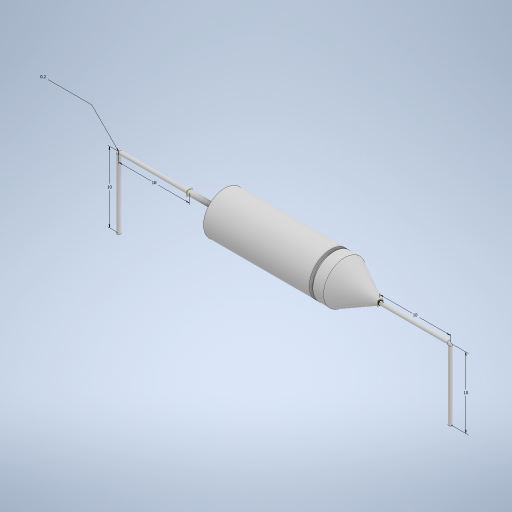
# Autodesk Inventor part: k50-29
Saved by Autodesk Inventor 2024 (Build 280153000, 153)
## iProperties
Created: 2023-12-15
Part Number: k50-29
Material: Generic
Document SubType Name: Sheet Metal
Designer: user
Density: 1 g/cm^3
Sheet Metal Rule: Default
Appearance: Default
Author: user
Autodesk Inventor part; units mm, degrees
ref_plane "YZ Plane" through (0, 0, 0) normal (1, 0, 0) x (0, 1, 0)
ref_plane "XZ Plane" through (0, 0, 0) normal (0, 1, 0) x (-1, 0, 0)
ref_plane "XY Plane" through (0, 0, 0) normal (0, 0, 1) x (1, 0, 0)
sketch "Sketch1" plane through (0, 0, 0) normal (0, 0, 1) x (1, 0, 0)
  line L0 (0, 0) -> (0, 0.35)
  line L1 (0, 0.35) -> (5, 0.35)
  line L2 (5, 0.35) -> (5, 3)
  line L3 (5, 3) -> (20, 3)
  line L4 (20, 3) -> (20, 2.5)
  line L5 (20, 2.5) -> (20.5, 2.5)
  line L6 (20.5, 2.5) -> (20.5, 3)
  line L7 (20.5, 3) -> (22, 3)
  line L8 (0, 0) -> (27, 0)
  line L9 (27, 0) -> (27, 0.35)
  line L10 (27, 0.35) -> (22, 3)
  dimension "d0" = 0.35
  dimension "d1" = 5
  dimension "d2" = 2.65
  dimension "d3" = 15
  dimension "d4" = 0.5
  dimension "d5" = 0.5
  dimension "d6" = 0.5
  dimension "d7" = 1.5
  dimension "d8" = 27
  dimension "d9" = 0.35
  constraints: 22 end point, 6 perpendicular, 2 point on line, 1 horizontal, 1 vertical
  measures "d0" distance of L0.start L0.end
  measures "d1" distance of L0.end L1.end
  measures "d2" distance of L1.end L2.end
  measures "d3" distance of L2.end L3.end
  measures "d4" distance of L3.end L4.end
  measures "d5" distance of L4.end L5.end
  measures "d6" distance of L5.end L6.end
  measures "d7" distance of L6.end L7.end
  measures "d8" distance of L0.start L8.end
  measures "d9" distance of L8.end L9.end
revolve "Revolution1" add sketch "Sketch1" angle 360 about axis through (0, 0, 0) along (1, 0, 0)
ref_plane "Work Plane1" through (27, 0, 0) normal (1, 0, 0) x (0, 0, -1)
sketch "Sketch2" plane through (27, 0, 0) normal (1, 0, 0) x (0, 0, -1)
  circle A0 centre (0, 0) radius 0.25
  dimension "d12" = 0.5
  constraints: 1 centre point, 1 coincident
  measures "d12" diameter of A0
ref_plane "Work Plane2" through (0, 0, 0) normal (-1, 0, 0) x (0, 0, 1)
sketch "Sketch3" plane through (0, 0, 0) normal (-1, 0, 0) x (0, 0, 1)
  circle A0 centre (0, 0) radius 0.25
  dimension "d14" = 0.5
  constraints: 1 centre point, 1 coincident
  measures "d14" diameter of A0
sketch "Sketch4" plane through (0, 0, 0) normal (0, 0, 1) x (1, 0, 0)
  line L0 (0, 0) -> (-9.8, 0)
  line L1 (-10, -0.2) -> (-10, -10)
  line L2 (26.9718, 0) -> (36.7718, 0)
  line L3 (36.9718, -0.2) -> (36.9718, -10)
  arc A0 (-9.8, 0) -> (-10, -0.2) centre (-9.8, -0.2) ccw
  arc A1 (36.9718, -0.2) -> (36.7718, 0) centre (36.7718, -0.2) ccw
  point P0 (-10, 0)
  point P1 (36.9718, 0)
  dimension "d15" = 10
  dimension "d16" = 10
  dimension "d17" = 10
  dimension "d18" = 10
  dimension "d19" = 0.2
  constraints: 8 end point, 4 point on circle, 4 point on line, 4 tangent, 2 centre point, 2 horizontal, 2 perpendicular, 1 equal radius
  measures "d15" distance of L0.start point (-10, 0)
  measures "d16" distance of point (-10, 0) L1.end
  measures "d17" distance of L2.start point (36.972, 0)
  measures "d18" distance of point (36.972, 0) L3.end
  measures "d19" radius of A0
sweep "Sweep1" add profiles "Sketch2" path "Sketch4" path curves L2 A1 L3
sweep "Sweep2" add profiles "Sketch3" path "Sketch4" path curves L0 A0 L1
equation "\"BendRadius\" = Thickness"
equation "\"BendReliefWidth\" = Thickness"
equation "\"BendReliefDepth\" = 0.5 * Thickness"
equation "\"CornerReliefSize\" = 4 * Thickness"
equation "\"MinimumRemnant\" = 2 * Thickness"
equation "\"TransitionRadius\" = BendRadius"
equation "\"JacobiRadiusSize\" = BendRadius"
equation "\"GapSize\" = Thickness"
equation "\"Thickness\" = 3.048"
body "Solid1"
